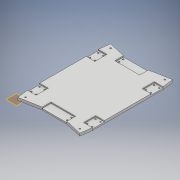
# Autodesk Inventor part: 3枚目
Saved by Autodesk Inventor 2018 (Build 220112000, 112)
## iProperties
Created: 2018-08-16
Part Number: 3枚目
Material: 一般
Document SubType Name: Modeling
Designer: shun2
Density: 1 g/cm^3
Appearance: 既定
Author: shun2
Autodesk Inventor part; units mm, degrees
ref_plane "YZ Plane" through (0, 0, 0) normal (1, 0, 0) x (0, 1, 0)
ref_plane "XZ Plane" through (0, 0, 0) normal (0, 1, 0) x (-1, 0, 0)
ref_plane "XY Plane" through (0, 0, 0) normal (0, 0, 1) x (1, 0, 0)
ref_plane "作業平面1" through (0, 0, 5.5) normal (0, 0, 1) x (1, 0, 0)
sketch "スケッチ3" plane through (0, 0, 5.5) normal (0, 0, 1) x (1, 0, 0)
  line L0 (0, 171.7239) -> (0, 23)
  line L1 (0, 23) -> (3, 0)
  line L2 (136, 23) -> (136, 171.7239)
  line L3 (136, 171.7239) -> (133.0079, 194.6636)
  line L4 (0, 23) -> (0, 75)
  line L5 (0, 127.7239) -> (0, 171.7239)
  line L6 (136, 171.7239) -> (136, 119.7239)
  line L7 (136, 67) -> (136, 23)
  circle A0 centre (11, 186.7239) radius 1.6
  circle A1 centre (125, 186.7239) radius 1.6
  circle A2 centre (11, 8) radius 1.6
  circle A3 centre (125, 8) radius 1.6
  line L8 (6.4, 186.7239) -> (15.6, 186.7239)
  line L9 (11, 182.1239) -> (11, 191.3239)
  line L10 (120.4, 186.7239) -> (129.6, 186.7239)
  line L11 (125, 182.1239) -> (125, 191.3239)
  line L12 (6.4, 8) -> (15.6, 8)
  line L13 (11, 3.4) -> (11, 12.6)
  line L14 (120.4, 8) -> (129.6, 8)
  line L15 (0, 127.7239) -> (0, 171.7239)
  line L16 (136, 171.7239) -> (136, 119.7239)
  line L17 (136, 67) -> (136, 23)
  line L18 (0, 23) -> (0, 75)
  line L19 (0, 171.7239) -> (3, 194.7239)
  line L20 (133, 0) -> (136, 23)
  line L21 (136, 46) -> (136, 23)
  line L22 (136, 23) -> (117.7, 23)
  line L23 (117.7, 23) -> (117.7, 48.5)
  line L24 (117.7, 48.5) -> (136, 48.5)
  line L25 (136, 48.5) -> (136, 23)
  line L26 (0, 23) -> (18.3, 23)
  line L27 (18.3, 23) -> (18.3, 48.5)
  line L28 (18.3, 48.5) -> (0, 48.5)
  line L29 (0, 48.5) -> (0, 23)
  line L30 (136, 171.7239) -> (117.7, 171.7239)
  line L31 (117.7, 171.7239) -> (117.7, 146.2239)
  line L32 (117.7, 146.2239) -> (136, 146.2239)
  line L33 (136, 146.2239) -> (136, 171.7239)
  line L34 (0, 171.7239) -> (18.3, 171.7239)
  line L35 (18.3, 171.7239) -> (18.3, 146.2239)
  line L36 (18.3, 146.2239) -> (0, 146.2239)
  line L37 (0, 146.2239) -> (0, 171.7239)
  circle A4 centre (132, 27) radius 1.6
  circle A5 centre (121.2, 27) radius 1.6
  circle A6 centre (132, 44.5) radius 1.6
  circle A7 centre (121.2, 44.5) radius 1.6
  circle A8 centre (132, 150.2239) radius 1.6
  circle A9 centre (132, 167.7239) radius 1.6
  circle A10 centre (121.2, 150.2239) radius 1.6
  circle A11 centre (121.2, 167.7239) radius 1.6
  circle A12 centre (14.8, 27) radius 1.6
  circle A13 centre (4, 27) radius 1.6
  circle A14 centre (14.8, 44.5) radius 1.6
  circle A15 centre (4, 44.5) radius 1.6
  circle A16 centre (14.8, 150.2239) radius 1.6
  circle A17 centre (4, 150.2239) radius 1.6
  circle A18 centre (14.8, 167.7239) radius 1.6
  circle A19 centre (4, 167.7239) radius 1.6
  line L38 (3, 194.7239) -> (38, 186.7239)
  line L39 (90.1667, 186.7239) -> (133.0079, 194.6636)
  line L40 (98, 8) -> (133, 0)
  line L41 (46.1667, 8) -> (3, 0)
  line L42 (90.1667, 186.7239) -> (38, 186.7239)
  line L43 (38, 186.7239) -> (38, 168.4239)
  line L44 (38, 168.4239) -> (90.1667, 168.4239)
  line L45 (90.1667, 168.4239) -> (90.1667, 186.7239)
  line L46 (98, 8) -> (46.1667, 8)
  line L47 (46.1667, 8) -> (46.1667, 26.3)
  line L48 (46.1667, 26.3) -> (98, 26.3)
  line L49 (98, 26.3) -> (98, 8)
  circle A20 centre (94, 12.65) radius 1.6
  circle A21 centre (94, 21.65) radius 1.6
  circle A22 centre (42, 173.0739) radius 1.6
  circle A23 centre (42, 182.0739) radius 1.6
  point P0 (0, 0)
  point P1 (0, 179.7239)
  dimension "d133" = 18.3
  dimension "d134" = 18.3
  dimension "d137" = 3.2
  dimension "d139" = 3.2
  constraints: 100 end point, 24 centre point, 14 parallel, 6 horizontal, 6 perpendicular, 2 point on line
  measures "d133" distance of L43.end L42.end
  measures "d134" distance of L46.end L47.end
  measures "d137" diameter of A20
  measures "d139" diameter of A21
ref_plane "作業平面6" through (0, 0, 5.5) normal (0, 0, 1) x (1, 0, 0)
extrude "押し出し8" add sketch "スケッチ3" along normal blind 3 contours L34 L35 L36 L0 | L42 L45 L44 L43 | L28 L27 L26 L0 | L2 L32 L31 L30 | L47 L48 L49 L46 | L2 L22 L23 L24
sketch "スケッチ9" plane through (0, 0, 5.5) normal (0, 0, -1) x (-1, 0, 0)
  line L0 (0, 146.2239) -> (0, 48.5)
  line L1 (0, 48.5) -> (0, 75)
  line L2 (0, 127.7239) -> (0, 146.2239)
  line L3 (0, 127.7239) -> (0, 146.2239)
  line L4 (0, 48.5) -> (0, 75)
  line L5 (-136, 171.7239) -> (-133.0079, 194.6636)
  circle A0 centre (-11, 186.7239) radius 1.6
  circle A1 centre (-125, 186.7239) radius 1.6
  circle A2 centre (-11, 8) radius 1.6
  circle A3 centre (-125, 8) radius 1.6
  line L6 (-6.4, 186.7239) -> (-15.6, 186.7239)
  line L7 (-11, 182.1239) -> (-11, 191.3239)
  line L8 (-120.4, 186.7239) -> (-129.6, 186.7239)
  line L9 (-125, 182.1239) -> (-125, 191.3239)
  line L10 (-6.4, 8) -> (-15.6, 8)
  line L11 (-11, 3.4) -> (-11, 12.6)
  line L12 (-120.4, 8) -> (-129.6, 8)
  line L13 (-133, 0) -> (-136, 23)
  line L14 (-136, 23) -> (-117.7, 23)
  line L15 (-117.7, 23) -> (-117.7, 48.5)
  line L16 (-117.7, 48.5) -> (-136, 48.5)
  line L17 (0, 23) -> (-18.3, 23)
  line L18 (-18.3, 23) -> (-18.3, 48.5)
  line L19 (-18.3, 48.5) -> (0, 48.5)
  line L20 (-117.7, 171.7239) -> (-117.7, 146.2239)
  line L21 (-117.7, 146.2239) -> (-136, 146.2239)
  circle A4 centre (-132, 27) radius 1.6
  circle A5 centre (-121.2, 27) radius 1.6
  circle A6 centre (-132, 44.5) radius 1.6
  circle A7 centre (-121.2, 44.5) radius 1.6
  circle A8 centre (-132, 150.2239) radius 1.6
  circle A9 centre (-132, 167.7239) radius 1.6
  circle A10 centre (-121.2, 150.2239) radius 1.6
  circle A11 centre (-121.2, 167.7239) radius 1.6
  circle A12 centre (-14.8, 27) radius 1.6
  circle A13 centre (-4, 27) radius 1.6
  circle A14 centre (-14.8, 44.5) radius 1.6
  circle A15 centre (-4, 44.5) radius 1.6
  line L22 (-90.1667, 186.7239) -> (-133.0079, 194.6636)
  line L23 (-98, 8) -> (-133, 0)
  line L24 (-46.1667, 8) -> (-3, 0)
  line L25 (-46.1667, 26.3) -> (-98, 26.3)
  line L26 (-98, 26.3) -> (-98, 8)
  circle A16 centre (-94, 12.65) radius 1.6
  circle A17 centre (-94, 21.65) radius 1.6
  circle A18 centre (-4, 150.2239) radius 1.6
  circle A19 centre (-14.8, 150.2239) radius 1.6
  circle A20 centre (-4, 167.7239) radius 1.6
  circle A21 centre (-14.8, 167.7239) radius 1.6
  circle A22 centre (-42, 173.0739) radius 1.6 projected
  circle A23 centre (-42, 173.0739) radius 1.6
  circle A24 centre (-42, 182.0739) radius 1.6 projected
  circle A25 centre (-42, 182.0739) radius 1.6
  line L27 (-38, 186.7239) -> (-38, 168.4239) projected
  line L28 (-90.1667, 168.4239) -> (-90.1667, 186.7239) projected
  line L29 (-38, 168.4239) -> (-90.1667, 168.4239)
  line L30 (-90.1667, 168.4239) -> (-90.1667, 186.7239)
  line L31 (-38, 186.7239) -> (-38, 168.4239)
  line L32 (0, 0) -> (0, 23) construction
  line L33 (-136, 171.7239) -> (-117.7, 171.7239) projected
  line L34 (-117.7, 171.7239) -> (-136, 171.7239)
  line L35 (0, 48.5) -> (0, 146.2239) construction
  line L36 (0, 171.7239) -> (0, 236.1886) construction
  line L37 (-38, 186.7239) -> (-3, 194.7239)
  line L38 (0, 171.7239) -> (-3, 194.7239)
  line L39 (-18.3, 146.2239) -> (0, 146.2239)
  line L40 (-18.3, 171.7239) -> (-18.3, 146.2239)
  line L41 (-18.3, 146.2239) -> (0, 146.2239)
  line L42 (-18.3, 171.7239) -> (0, 171.7239) projected
  line L43 (0, 171.7239) -> (-18.3, 171.7239)
  line L44 (-136, 48.5) -> (-136, 146.2239)
  line L45 (-46.1667, 8) -> (-46.1667, 26.3)
  line L46 (0, 23) -> (-18.3, 23) projected
  line L47 (-3, 0) -> (0, 23)
  point P0 (0, 179.7239)
  dimension "d150" = 3.2
  dimension "d151" = 3.2
  dimension "d152" = 3.2
  dimension "d153" = 3.2
  dimension "d154" = 3.2
  dimension "d155" = 3.2
  constraints: 86 end point, 24 centre point, 5 vertical, 2 coincident, 2 equal length, 2 horizontal, 2 perpendicular, 1 point on line, 1 other
  measures "d150" diameter of A18
  measures "d151" diameter of A19
  measures "d152" diameter of A20
  measures "d153" diameter of A21
  measures "d154" diameter of A23
  measures "d155" diameter of A25
extrude "押し出し9" add sketch "スケッチ9" against normal blind 5.5 contours L0 L19 L18 L17 L47 L24 L45 L25 L26 L23 L13 L14 L15 L16 L44 L21 L20 L33 L5 L22 L28 L29 L27 L37 L38 L42 L40 L39
